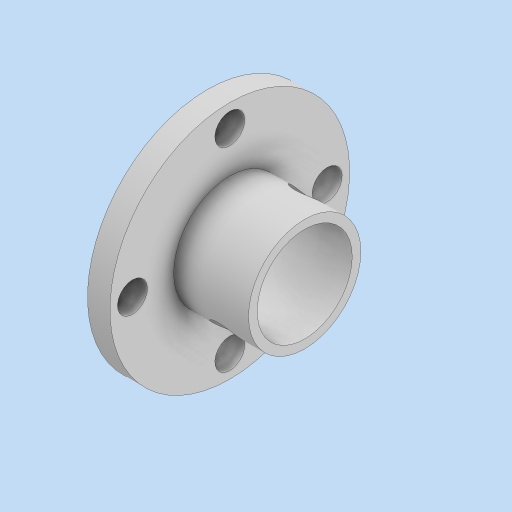
# Autodesk Inventor part: HipCoupler
Saved by Autodesk Inventor 2024 (Build 280153000, 153)
## iProperties
Created: 2023-10-20
Part Number: HipCoupler
Material: Generic
Document SubType Name: Modeling
Designer: megan
Density: 1 g/cm^3
Appearance: Default
Author: megan
Autodesk Inventor part; units mm, degrees
ref_plane "YZ Plane" through (0, 0, 0) normal (1, 0, 0) x (0, 1, 0)
sketch "Sketch1" plane through (0, 0, 0) normal (1, 0, 0) x (0, 1, 0)
  circle A0 centre (0, 0) radius 16
  circle A1 centre (0, 13) radius 2
  circle A2 centre (0, -13) radius 2
  circle A3 centre (-13, 0) radius 2
  circle A4 centre (13, 0) radius 2
  circle A5 centre (0, -13) radius 2
  circle A6 centre (0, 13) radius 2
  circle A7 centre (13, 0) radius 2
  circle A8 centre (-13, 0) radius 2
  circle A9 centre (0, 0) radius 6.35
  line L0 (0, -22.4) -> (0, 22.4) projected
  dimension "d0" = 32
  dimension "d1" = 4
  dimension "d2" = 26
  dimension "d3" = 13
  dimension "d6" = 360
  dimension "d8" = 12.7
  constraints: 10 centre point, 2 coincident, 1 equal radius, 17 other
  measures "d0" diameter of A0
  measures "d1" diameter of A1
  measures "d2" distance of A2.centre A1.centre
  measures "d3" distance of point (0, 0) A2.centre
  measures "d8" diameter of A9
extrude "Extrusion1" add sketch "Sketch1" along normal blind 3 contours A0 L0 A2 A9 A1 | L0 A1 A9 A2 A0
sketch "Sketch2" plane through (3, 0, 0) normal (1, 0, 0) x (0, 0, -1)
  circle A0 centre (0, 0) radius 16 projected
  circle A1 centre (13, 0) radius 2 projected
  circle A2 centre (0, 0) radius 6.35 projected
  circle A3 centre (0, -13) radius 2 projected
  circle A4 centre (-13, 0) radius 2 projected
  circle A5 centre (0, 13) radius 2 projected
  circle A6 centre (0, 0) radius 7.5
  dimension "d11" = 15
  constraints: 1 centre point, 1 coincident
  measures "d11" diameter of A6
extrude "Extrusion2" add sketch "Sketch2" along normal blind 10 contours A6
ref_plane "Work Plane1" through (0, 0, 0) normal (0, 0.7071, -0.7071) x (-1, 0, 0)
sketch "Sketch5" plane through (0, 0, 0) normal (0, 0.7071, -0.7071) x (-1, 0, 0)
  circle A0 centre (-8, 0) radius 2
  line L0 (-13, 7.5) -> (-13, -7.5) projected
  line L1 (-3, -7.5) -> (-3, 7.5) projected
  point P0 (0, 0)
  point P1 (-13, 0)
  dimension "d14" = 4
  dimension "d15" = 5
  constraints: 1 centre point, 1 midpoint
  measures "d14" diameter of A0
  measures "d15" distance of point (-13, 0) A0.centre
extrude "Extrusion3" cut sketch "Sketch5" along normal through all both and the other way through all
body "Solid1"
